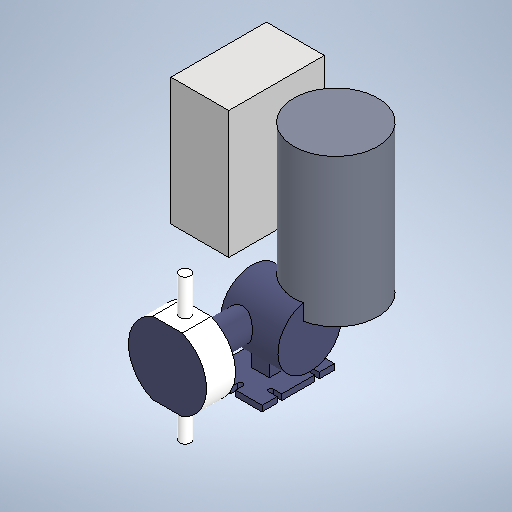
# Autodesk Inventor part: Spring MS1 Elektra
Saved by Autodesk Inventor 2025.1 (Build 291241020, 241B)
## iProperties
Created: 2024-11-03
Part Number: Spring MS1 Elektra
Material: Generic
Document SubType Name: Modeling
Designer: admin
Density: 1 g/cm^3
Appearance: Default
Author: admin
Autodesk Inventor part; units mm, degrees
ref_plane "YZ Plane" through (0, 0, 0) normal (1, 0, 0) x (0, 1, 0)
ref_plane "XZ Plane" through (0, 0, 0) normal (0, 1, 0) x (-1, 0, 0)
sketch "Sketch1" plane through (0, 0, 0) normal (0, 0, 1) x (1, 0, 0)
  line L0 (-50, 62.5) -> (50, 62.5)
  line L1 (50, 62.5) -> (50, -62.5)
  line L2 (50, -62.5) -> (-50, -62.5)
  line L3 (-50, -62.5) -> (-50, 62.5)
  line L4 (-50, 62.5) -> (50, -62.5) construction
  line L5 (50, 62.5) -> (-50, -62.5) construction
  line L6 (50, 36.5) -> (35, 36.5)
  arc A0 (35, 36.5) -> (35, 28.5) centre (35, 32.5) ccw
  line L7 (35, 28.5) -> (50, 28.5)
  line L8 (50, -28.5) -> (35, -28.5)
  arc A1 (35, -28.5) -> (35, -36.5) centre (35, -32.5) ccw
  line L9 (35, -36.5) -> (50, -36.5)
  line L10 (4.5, 62.5) -> (4.5, 50)
  arc A2 (-4.5, 50) -> (4.5, 50) centre (0, 50) ccw
  line L11 (-4.5, 50) -> (-4.5, 62.5)
  line L12 (4.5, -62.5) -> (4.5, -50)
  arc A3 (4.5, -50) -> (-4.5, -50) centre (0, -50) ccw
  line L13 (-4.5, -50) -> (-4.5, -62.5)
  line L14 (-50, -36.5) -> (-35, -36.5)
  arc A4 (-35, -36.5) -> (-35, -28.5) centre (-35, -32.5) ccw
  line L15 (-35, -28.5) -> (-50, -28.5)
  line L16 (-50, 28.5) -> (-35, 28.5)
  arc A5 (-35, 28.5) -> (-35, 36.5) centre (-35, 32.5) ccw
  line L17 (-35, 36.5) -> (-50, 36.5)
  line L18 (50, 0) -> (-50, 0) construction
  point P0 (0, 0)
  point P1 (0, 0)
  dimension "d0" = 100
  dimension "d1" = 125
  dimension "d2" = 4
  dimension "d3" = 65
  dimension "d4" = 15
  dimension "d5" = 4.5
  dimension "d6" = 12.5
  dimension "d39" = 70
  dimension "d40" = 100
  constraints: 38 end point, 16 point on line, 12 point on circle, 11 tangent, 9 perpendicular, 6 centre point, 5 midpoint, 4 equal length, 4 equal radius, 2 horizontal, 2 parallel, 2 vertical alignment, 1 horizontal alignment, 1 vertical, 1 other
  measures "d0" distance of L1.end L2.end
  measures "d1" distance of L0.end L1.end
  measures "d2" radius of A0
  measures "d3" distance of A1.centre A0.centre
  measures "d4" distance from line of L1 A0.centre
  measures "d5" radius of A2
  measures "d6" distance of L11.start L11.end
  measures "d39" distance of A1.centre A4.centre
  measures "d40" distance of A3.centre A2.centre
extrude "Extrusion1" add sketch "Sketch1" along normal blind 10 contours L0 L11 A2 L10 L1 L6 A0 L7 L8 A1 L9 L2 L12 A3 L13 L3 L14 A4 L15 L16 A5 L17
sketch "Sketch3" plane through (0, 0, 0) normal (0, 0, 1) x (1, 0, 0)
  line L0 (-15, 35) -> (15, 35)
  line L1 (15, 35) -> (15, -15)
  line L2 (15, -15) -> (-15, -15)
  line L3 (-15, -15) -> (-15, 35)
  point P0 (0, 0)
  point P1 (0, -15)
  dimension "d9" = 30
  dimension "d10" = 50
  dimension "d11" = 15
  constraints: 8 end point, 2 parallel, 1 horizontal, 1 midpoint, 1 perpendicular, 1 vertical alignment
  measures "d9" distance of L0.start L0.end
  measures "d10" distance of L2.end L0.start
  measures "d11" distance from line of point (0, 0) L2
extrude "Extrusion2" add sketch "Sketch3" along normal blind 120
sketch "Sketch4" plane through (0, 0, 0) normal (1, 0, 0) x (0, 1, 0)
  circle A0 centre (0, 94) radius 55
  line L0 (28.5, 0) -> (-28.5, 0) projected
  point P0 (0, 0)
  point P1 (0, 0)
  point P2 (0, 0)
  dimension "d14" = 94
  dimension "d15" = 110
  dimension "d16" = 0
  constraints: 2 midpoint, 1 centre point
  measures "d14" distance of point (0, 0) A0.centre
  measures "d15" diameter of A0
  measures "d16" horizontal distance of point (0, 0) A0.centre
extrude "Extrusion3" add sketch "Sketch4" along normal blind 70 and the other way blind 30
sketch "Sketch5" plane through (0, 0, 120) normal (0, 0, 1) x (1, 0, 0)
  circle A0 centre (55, 60) radius 72.5
  point P0 (0, 0)
  dimension "d21" = 145
  dimension "d22" = 55
  dimension "d23" = 60
  constraints: 1 centre point
  measures "d21" diameter of A0
  measures "d22" horizontal distance of A0.centre point (0, 0)
  measures "d23" vertical distance of A0.centre point (0, 0)
extrude "Extrusion4" add sketch "Sketch5" along normal blind 255
sketch "Sketch6" plane through (0, 0, 0) normal (0, 1, 0) x (-1, 0, 0)
  circle A0 centre (0, 100) radius 25
  point P0 (0, 0)
  dimension "d26" = 50
  dimension "d27" = 100
  constraints: 1 centre point, 1 vertical alignment
  measures "d26" diameter of A0
  measures "d27" distance of A0.centre point (0, 0)
extrude "Extrusion5" add sketch "Sketch6" against normal blind 176
sketch "Sketch7" plane through (0, -176, 100) normal (0, -1, 0) x (1, 0, 0)
  circle A0 centre (0, 0) radius 67.5
  line L0 (-25.4951, 62.5) -> (25.4951, 62.5)
  line L1 (-25.4951, -62.5) -> (25.4951, -62.5)
  circle A1 centre (0, 0) radius 25 construction
  line L2 (0, 0) -> (67.5, 0) construction
  point P0 (0, -100)
  dimension "d30" = 135
  dimension "d31" = 125
  constraints: 6 end point, 5 point on circle, 3 horizontal, 1 centre point, 1 coincident, 1 other
  measures "d30" diameter of A0
  measures "d31" distance between parallel lines of L1 L0
extrude "Extrusion6" add sketch "Sketch7" against normal blind 50 contours A0 L1 L0
ref_plane "Work Plane1" through (0, 0, 100) normal (0, 0, 1) x (1, 0, 0)
sketch "Sketch8" plane through (0, 0, 100) normal (0, 0, 1) x (1, 0, 0)
  circle A0 centre (0, -145.5) radius 9.525
  point P0 (0, 0)
  dimension "d35" = 19.05
  dimension "d36" = 145.5
  constraints: 1 centre point, 1 vertical alignment
  measures "d35" diameter of A0
  measures "d36" distance of point (0, 0) A0.centre
extrude "Extrusion7" add sketch "Sketch8" along normal mid plane 250
sketch "Sketch9" plane through (-30, 0, 94) normal (-1, 0, 0) x (0, 0, 1)
  line L0 (306, 125) -> (86, 125)
  line L1 (86, 125) -> (86, -40)
  line L2 (86, -40) -> (306, -40)
  line L3 (306, -40) -> (306, 125)
  line L4 (-94, 28.5) -> (-94, -28.5) projected
  point P0 (-94, 0)
  point P1 (-94, 0)
  point P2 (-94, 0)
  dimension "d41" = 165
  dimension "d42" = 220
  dimension "d43" = 180
  dimension "d44" = 40
  constraints: 8 end point, 2 midpoint, 2 parallel, 1 horizontal, 1 perpendicular
  measures "d41" distance of L2.end L0.start
  measures "d42" distance of L1.end L2.end
  measures "d43" distance from line of point (-94, 0) L1
  measures "d44" distance from line of L2 point (-94, 0)
extrude "Extrusion8" add sketch "Sketch9" along normal blind 100
body "Solid1"
